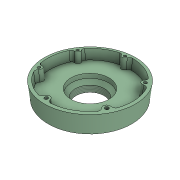
# Autodesk Inventor part: Cap Housing Base
Saved by Autodesk Inventor 2020.1 (Build 241239000, 239)
## iProperties
Created: 2019-11-13
Part Number: Cap Housing Base
Material: Generic
Document SubType Name: Modeling
Designer: thom_tremblay
Density: 1 g/cm^3
Appearance: Rubber - Green
Author: thom_tremblay
Autodesk Inventor part; units mm, degrees
ref_plane "YZ Plane" through (0, 0, 0) normal (1, 0, 0) x (0, 1, 0)
ref_plane "XZ Plane" through (0, 0, 0) normal (0, 1, 0) x (-1, 0, 0)
ref_plane "XY Plane" through (0, 0, 0) normal (0, 0, 1) x (1, 0, 0)
sketch "Sketch1" plane through (0, 0, 0) normal (0, 0, 1) x (1, 0, 0)
  line L0 (71.12, 17.78) -> (66.548, 17.78)
  line L1 (66.548, 17.78) -> (66.548, -7.62)
  line L2 (66.548, -7.62) -> (71.12, -7.62)
  line L3 (71.12, -7.62) -> (71.12, 17.78)
  line L4 (66.548, -7.62) -> (31.75, -7.62)
  line L5 (31.75, -7.62) -> (31.75, 0)
  line L6 (31.75, 0) -> (66.548, 0)
  line L7 (66.548, 0) -> (66.548, -7.62)
  line L8 (25.4, -13.97) -> (30.48, -13.97)
  line L9 (30.48, -13.97) -> (30.48, -25.4)
  line L10 (30.48, -25.4) -> (25.4, -25.4)
  line L11 (25.4, -25.4) -> (25.4, -13.97)
  line L12 (0, 0) -> (0, -50.8709) construction
  line L13 (25.4, -13.97) -> (31.75, -7.62)
  line L14 (30.48, -13.97) -> (36.83, -7.62)
  dimension "d0" = 142.24
  dimension "d1" = 50.8
  dimension "d2" = 4.572
  dimension "d4" = 6.35
  dimension "d5" = 11.43
  dimension "d6" = 25.4
  dimension "d7" = 45
  dimension "d9" = 5.08
  dimension "d10" = 7.62
  constraints: 30 end point, 9 perpendicular, 2 horizontal, 2 point on line, 1 parallel
  measures "d0" diameter of L3 L12
  measures "d1" diameter of L11 L12
  measures "d2" distance of L0.start L0.end
  measures "d4" distance between parallel lines of L5 L11
  measures "d5" distance of L10.end L8.start
  measures "d6" distance of L2.end L0.start
  measures "d7" angle of L9 L13
  measures "d9" distance of L9.end L10.end
  measures "d10" distance of L4.end L5.end
revolve "Revolution1" add sketch "Sketch1" angle 360 about axis through (0, 0, 0) along (0, -1, 0)
sketch "Sketch2" plane through (0, 17.78, 0) normal (0, 1, 0) x (1, 0, 0)
  circle A0 centre (0, 0) radius 71.12 projected
  line L0 (0, 0) -> (0, 63.5) construction
  circle A1 centre (0, 63.5) radius 5.08
  dimension "d11" = 63.5
  dimension "d12" = 10.16
  constraints: 2 end point, 1 centre point, 1 coincident, 1 vertical
  measures "d11" distance of L0.start L0.end
  measures "d12" diameter of A1
extrude "Extrusion1" add sketch "Sketch2" against normal up to surface (17.78 mm away) contours A1
fillet "Fillet1" radius 5.08 2 edges at (4.1584, 8.89, -66.418) (-4.1584, 8.89, -66.418)
pattern_circular "Circular Pattern1" count 6 over 360 about axis through (0, -19.685, 0) along (0, -1, 0) of "Extrusion1", "Fillet1"
thread "Thread1" size "2" designation "2 - 11.5 NPT" standard "NPT" length 26.8732
sketch "Sketch3" plane through (0, 17.78, 0) normal (0, 1, 0) x (1, 0, 0)
  arc A0 (-4.8815, 62.0939) -> (4.8815, 62.0939) centre (0, 63.5) ccw projected
  arc A1 (-51.3341, -35.2744) -> (-56.2156, -26.8194) centre (-54.9926, -31.75) ccw projected
  arc A2 (4.8815, -62.0939) -> (-4.8815, -62.0939) centre (0, -63.5) ccw projected
  arc A3 (56.2156, -26.8194) -> (51.3341, -35.2744) centre (54.9926, -31.75) ccw projected
  arc A4 (51.3341, 35.2744) -> (56.2156, 26.8194) centre (54.9926, 31.75) ccw projected
  arc A5 (-56.2156, 26.8194) -> (-51.3341, 35.2744) centre (-54.9926, 31.75) ccw projected
  point P0 (0, 63.5)
  point P1 (-51.8006, -35.7019)
  point P2 (-56.819, -27.0097)
  point P3 (5.0184, -62.7116)
  point P4 (-5.0184, -62.7116)
  point P5 (56.819, -27.0097)
  point P6 (51.8006, -35.7019)
  point P7 (51.8006, 35.7019)
  point P8 (56.819, 27.0097)
  point P9 (-56.819, 27.0097)
  point P10 (-51.8006, 35.7019)
  constraints: 6 coincident
hole "Hole1" at (0, 17.78, -63.5) at (-54.9926, 17.78, 31.75) at (0, 17.78, 63.5) at (54.9926, 17.78, 31.75) at (54.9926, 17.78, -31.75) at (-54.9926, 17.78, -31.75) direction (0, -1, 0) diameter 4.9784 depth 15.24 tip angle 118 thread size "1/4-20 UNC" class "2B" standard "ANSI Unified Screw Threads"
body "Solid1"
